9 Volt battery (Autodesk Fusion 360 design; units mm, degrees)
Autodesk Fusion 360 part; units mm, degrees
sketch "Sketch1" plane through (0, 0, 0) normal (0, 1, 0) x (1, 0, 0)
  line L0 (0, 0) -> (15, 0)
  line L1 (15, 0) -> (15, -25)
  line L2 (15, -25) -> (0, -25)
  line L3 (0, -25) -> (0, 0)
  dimension "d1" = 15
  dimension "d2" = 25
  constraint horizontal L0
  constraint vertical L1
  constraint horizontal L2
  constraint vertical L3
  constraint coincident L0.start L3.end
  measures "d1" distance of L0.start L0.end
  measures "d2" distance of L0.start L2.end
extrude "Extrude1" add sketch "Sketch1" along normal blind 48
sketch "Sketch2" plane through (0, 0, 0) normal (0, -1, 0) x (1, 0, 0)
  line L0 (15, 25) -> (0, 25)
  line L1 (0, 25) -> (0, 0)
  line L2 (0, 0) -> (15, 0)
  line L3 (15, 0) -> (15, 25)
  line L4 (5.4793, 22) -> (3.4585, 18.5)
  line L5 (3.4585, 18.5) -> (5.4793, 15)
  line L6 (5.4793, 15) -> (9.5207, 15)
  line L7 (9.5207, 15) -> (11.5415, 18.5)
  line L8 (11.5415, 18.5) -> (9.5207, 22)
  line L9 (9.5207, 22) -> (5.4793, 22)
  circle A0 centre (7.5, 6) radius 3.5
  point P0 (7.5, 18.5)
  dimension "d5" = 3.5
  dimension "d6" = 3
  dimension "d7" = 7.5
  dimension "d8" = 7
  dimension "d9" = 6
  dimension "d10" = 7.5
  constraint parallel L0 L9
  measures "d5" distance of P0 L9
  measures "d6" distance of L0 L9
  measures "d7" distance of L1 P0
  measures "d8" diameter of A0
  measures "d9" vertical distance of L1.end A0.centre
  measures "d10" horizontal distance of L1.end A0.centre
extrude "Extrude2" add sketch "Sketch2" along normal blind 3 contours L4 L5 L6 L7 L8 L9 | A0
move_body "Move1" bodies 1 to x (1, 0, 0) y (0, 0, -1) z (0, 1, 0) at (0, -3, -3)
move_body "Move2" bodies 1 to x (1, 0, 0) y (0, 1, 0) z (0, 0, 1) at (0, 0, 50)
move_body "Move3" bodies 1 to x (1, 0, 0) y (0, 1, 0) z (0, 0, 1) at (0, 0, 5)
move_body "Move4" bodies 1 to x (1, 0, 0) y (0, 0, 1) z (0, -1, 0) at (0, 1, 7)
move_body "Move5" bodies 1 to x (1, 0, 0) y (0, 1, 0) z (0, 0, 1) at (30, -25, 0)
